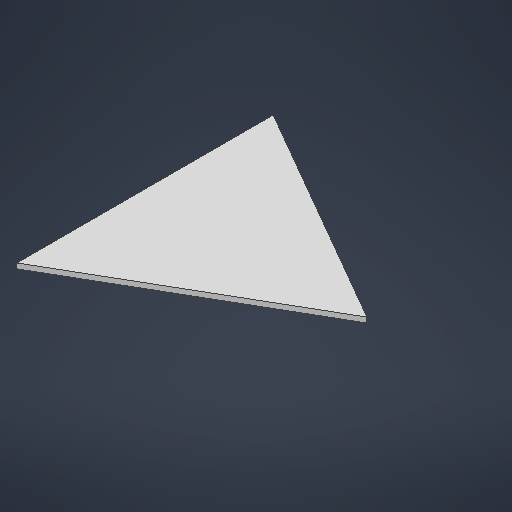
# Autodesk Inventor part: Pieza2
Saved by Autodesk Inventor 2027 (Build 310192060, 192F)
## iProperties
Created: 2026-08-23
Part Number: Pieza2
Material: Genérico
Document SubType Name: Modeling
Designer: Leandro
Density: 1 g/cm^3
Appearance: Valor por defecto
Author: Leandro
Autodesk Inventor part; units mm, degrees
ref_plane "YZ Plane" through (0, 0, 0) normal (1, 0, 0) x (0, 1, 0)
ref_plane "XZ Plane" through (0, 0, 0) normal (0, 1, 0) x (-1, 0, 0)
ref_plane "XY Plane" through (0, 0, 0) normal (0, 0, 1) x (1, 0, 0)
sketch "Boceto3" plane through (0, 0, 0) normal (0, 1, 0) x (-1, 0, 0)
  line L0 (-3.8363, 4.0581) -> (-3.8363, -95.9419)
  line L1 (-3.8363, -95.9419) -> (-90.4389, -45.9419)
  line L2 (-90.4389, -45.9419) -> (-3.8363, 4.0581)
  point P0 (0, 0)
  dimension "d7" = 100
  dimension "d8" = 100
  constraints: 6 end point, 1 vertical
  measures "d7" distance of L0.start L0.end
  measures "d8" distance of L0.end L1.end
extrude "Extrusión2" add sketch "Boceto3" along normal mid plane 2
